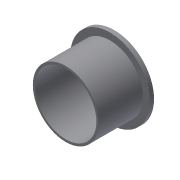
# Autodesk Inventor part: KuplungZar
Saved by Autodesk Inventor 2015 SP1 (Build 190203100, 203)
## iProperties
Created: 2015-04-15
Part Number: KuplungZar
Material: Generic
Document SubType Name: Modeling
Designer: laca
Density: 1 g/cm^3
Appearance: Default
Author: laca
Autodesk Inventor part; units mm, degrees
ref_plane "YZ Plane" through (0, 0, 0) normal (1, 0, 0) x (0, 1, 0)
ref_plane "XZ Plane" through (0, 0, 0) normal (0, 1, 0) x (-1, 0, 0)
sketch "Sketch1" plane through (0, 0, 0) normal (0, 0, 1) x (1, 0, 0)
  circle A0 centre (0, 0) radius 18.8718
  circle A1 centre (0, 0) radius 14.5325
  circle A2 centre (0, 0) radius 15.6226
  constraints: 3 centre point, 3 coincident
extrude "Extrusion1" add sketch "Sketch1" along normal blind 2 contours A0 | A2
ref_plane "Work Plane1" through (-29.0978, -29.0978, 23) normal (0, 0, -1) x (0, 1, 0)
extrude "Extrusion2" add sketch "Sketch1" along normal up to surface (23 mm away) contours A2
body "Solid1"
